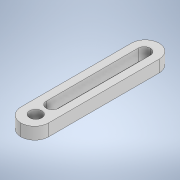
# Autodesk Inventor part: extention_plate
Saved by Autodesk Inventor 2020 (Build 240168000, 168)
## iProperties
Created: 2019-09-23
Part Number: extention_plate
Material: Generic
Document SubType Name: Modeling
Designer: dlr6513
Density: 1 g/cm^3
Appearance: Default
Author: dlr6513
Autodesk Inventor part; units mm, degrees
ref_plane "YZ Plane" through (0, 0, 0) normal (1, 0, 0) x (0, 1, 0)
ref_plane "XZ Plane" through (0, 0, 0) normal (0, 1, 0) x (-1, 0, 0)
ref_plane "XY Plane" through (0, 0, 0) normal (0, 0, 1) x (1, 0, 0)
sketch "Sketch1" plane through (0, 0, 0) normal (0, 1, 0) x (-1, 0, 0)
  line L0 (16.3851, 33.9368) -> (4.9404, 33.9368)
  line L1 (4.9404, 33.9368) -> (4.9404, -23.2869)
  line L2 (4.9404, -23.2869) -> (16.3851, -23.2869)
  line L3 (16.3851, -23.2869) -> (16.3851, 33.9368)
  line L4 (13.2127, 30.325) -> (8.1127, 30.325)
  line L5 (8.1127, 30.325) -> (8.1127, -19.675)
  line L6 (8.1127, -19.675) -> (13.2127, -19.675)
  line L7 (13.2127, -19.675) -> (13.2127, 30.325)
  circle A0 centre (10.6627, 27.775) radius 2.55
  line L8 (13.2127, 23.4447) -> (8.1127, 23.4447)
  point P0 (0, 0)
  dimension "d2" = 5.1
  dimension "d3" = 11.4447
  dimension "d4" = 57.2237
  dimension "d5" = 3.1724
  dimension "d6" = 50
  dimension "d7" = 3.6118
  dimension "d12" = 5.1
  dimension "d13" = 2.55
  constraints: 18 end point, 4 parallel, 3 perpendicular, 2 horizontal, 2 point on line, 1 centre point
  measures "d2" distance between parallel lines of L5 L7
  measures "d3" distance of L1.end L2.end
  measures "d4" distance of L2.end L0.start
  measures "d5" distance between parallel lines of L3 L7
  measures "d6" distance of L6.end L4.start
  measures "d7" distance between parallel lines of L0 L4
  measures "d12" diameter of A0
  measures "d13" distance from line of L4 A0.centre
extrude "Extrusion2" add sketch "Sketch1" along normal blind 5 contours L3 L2 L1 L0 | L7 A0 L4 | A0 L5 L4 | L7 L8 L5 A0
fillet "Fillet3" radius 5.715 4 edges at (-16.3851, 2.5, 33.9368) (-4.9404, 2.5, 33.9368) (-16.3851, 2.5, -23.2869) (-4.9404, 2.5, -23.2869)
fillet "Fillet4" radius 2.54 4 edges at (-13.2127, 2.5, 23.4447) (-8.1127, 2.5, 23.4447) (-8.1127, 2.5, -19.675) (-13.2127, 2.5, -19.675)
equation "\"d5\" = -0.5 * d2 + 0.5 * d3"
equation "\"d7\" = -0.5 * d6 + 0.5 * d4"
equation "\"d12\" = d2"
equation "\"d13\" = 0.5 * d2"
body "Solid2"
